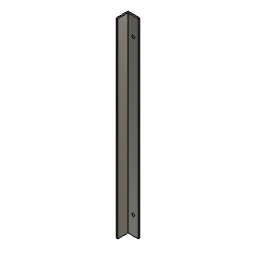
angle iron 1 inch 410 mm v5 (Autodesk Fusion 360 design; units mm, degrees)
Autodesk Fusion 360 part; units mm, degrees
sketch "Sketch1" plane through (0, 0, 0) normal (0, 0, 1) x (1, 0, 0)
  line L0 (0, 0) -> (25.4, 0)
  line L1 (0, 0) -> (0, -25.4)
  line L2 (3.175, -3.175) -> (25.4, -3.175)
  line L3 (3.175, -3.175) -> (3.175, -25.4)
  line L4 (25.4, 0) -> (25.4, -3.175)
  line L5 (0, -25.4) -> (3.175, -25.4)
  dimension "d1" = 25.4
  dimension "d2" = -3.175
  constraint coincident L0.start L1.start
  constraint horizontal L0
  constraint perpendicular L0 L1
  constraint equal L0 L1
  measures "d1" distance of L0.start L0.end
extrude "Extrude1" add sketch "Sketch1" along normal blind 410
sketch "Sketch2" plane through (0, -3.175, 0) normal (0, -1, 0) x (1, 0, 0)
  line L0 (3.175, 0) -> (25.4, 0)
  line L1 (25.4, 0) -> (25.4, 410)
  line L2 (25.4, 410) -> (3.175, 410)
  line L3 (3.175, 410) -> (3.175, 0)
  circle A0 centre (14.2875, 370.71) radius 4.4166
  circle A1 centre (14.2875, 39.29) radius 4.4166
  line L4 (14.2875, 410) -> (14.2875, 0) construction
  line L5 (14.2875, 205) -> (25.4, 205) construction
  dimension "d6" = 165.71
  dimension "d7" = 165.71
  constraint midpoint L2 L4.start
  constraint midpoint L0 L4.end
  constraint coincident A1.centre L4
  constraint coincident A0.centre L4
  constraint equal A0 A1
  constraint midpoint L4 L5.start
  constraint midpoint L1 L5.end
  measures "d6" distance of A1.centre L5.start
  measures "d7" distance of A0.centre L5.start
hole "Hole1" at (14.2875, -3.175, 370.71) at (14.2875, -3.175, 39.29) direction (0, 1, 0) diameter 5.5 depth 7 tip angle 118
